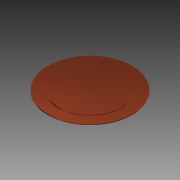
# Autodesk Inventor part: 12mmPiezo
Saved by Autodesk Inventor 2014 (Build 180170000, 170)
## iProperties
Created: 2014-10-12
Part Number: 12mmPiezo
Material: Generic
Document SubType Name: Modeling
Designer: DV
Density: 1 g/cm^3
Appearance: Default
Mass: 0.0189438 g
Surface Area: 2.33358 cm^2
Volume: 0.0189438 cm^3
Author: DV
Autodesk Inventor part; units mm, degrees
ref_plane "YZ Plane" through (0, 0, 0) normal (1, 0, 0) x (0, 1, 0)
ref_plane "XZ Plane" through (0, 0, 0) normal (0, 1, 0) x (-1, 0, 0)
ref_plane "XY Plane" through (0, 0, 0) normal (0, 0, 1) x (1, 0, 0)
sketch "Sketch1" plane through (0, 0, 0) normal (0, 0, 1) x (1, 0, 0)
  line L0 (0, 0) -> (6, 0)
  line L1 (6, 0) -> (6, 0.1)
  line L2 (6, 0.1) -> (0, 0.1)
  line L3 (0, 0.1) -> (0, 0)
  line L4 (0, 0.1) -> (4.5, 0.1)
  line L5 (4.5, 0.1) -> (4.5, 0.22)
  line L6 (4.5, 0.22) -> (0, 0.22)
  line L7 (0, 0.22) -> (0, 0.1)
  dimension "d0" = 6
  dimension "d1" = 0.1
  dimension "d2" = 4.5
  dimension "d3" = 0.12
  constraints: 16 end point, 4 parallel, 2 horizontal, 2 perpendicular
  measures "d0" distance of L2.end L1.end
  measures "d1" distance of L1.end L0.end
  measures "d2" distance of L6.end L5.end
  measures "d3" distance of L5.end L4.end
revolve "Revolution1" add sketch "Sketch1" angle 360 about axis through (0, 0.22, 0) along (0, -1, 0)
body "Solid1"
